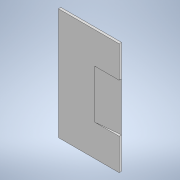
# Autodesk Inventor part: Stage
Saved by Autodesk Inventor 2021 (Build 250183000, 183)
## iProperties
Created: 2022-07-02
Part Number: Stage
Material: 一般
Document SubType Name: Modeling
Designer: tazak
Density: 1 g/cm^3
Appearance: 既定
Author: tazak
Autodesk Inventor part; units mm, degrees
ref_plane "YZ Plane" through (0, 0, 0) normal (1, 0, 0) x (0, 1, 0)
ref_plane "XZ Plane" through (0, 0, 0) normal (0, 1, 0) x (-1, 0, 0)
ref_plane "XY Plane" through (0, 0, 0) normal (0, 0, 1) x (1, 0, 0)
sketch "スケッチ1" plane through (0, 0, 0) normal (0, 0, 1) x (1, 0, 0)
  line L0 (-800, 2300) -> (1700, 2300)
  line L1 (1700, 2300) -> (1700, -2300)
  line L2 (1700, -2300) -> (-800, -2300)
  line L3 (-800, -2300) -> (-800, 2300)
  line L4 (-1000, 2500) -> (2000, 2500) construction
  line L5 (2000, 2500) -> (2000, -2500) construction
  line L6 (2000, -2500) -> (-1000, -2500) construction
  line L7 (-1000, -2500) -> (-1000, 2500) construction
  point P0 (0, 0)
  point P1 (-1000, 0)
  dimension "d13" = 2500
  dimension "d14" = 5000
  dimension "d15" = 1000
  dimension "d16" = 2000
  dimension "d17" = 200
  dimension "d18" = 200
  dimension "d19" = 200
  constraints: 16 end point, 4 parallel, 2 horizontal, 2 perpendicular, 1 horizontal alignment, 1 midpoint
  measures "d13" distance of L0.start L0.end
  measures "d14" distance of L6.end L4.start
  measures "d15" distance from line of point (0, 0) L7
  measures "d16" distance from line of L5 point (0, 0)
  measures "d17" distance between parallel lines of L3 L7
  measures "d18" distance between parallel lines of L4 L0
  measures "d19" distance between parallel lines of L6 L2
extrude "押し出し1" add sketch "スケッチ1" along normal blind 100
sketch "スケッチ4" plane through (0, 0, 0) normal (0, 1, 0) x (-1, 0, 0)
  line L0 (-1700, 0) -> (-700, 100)
  line L1 (-1700, 100) -> (800, 100) projected
  line L2 (-1700, 0) -> (-1700, 100) projected
  line L3 (-700, 100) -> (-1700, 100)
  line L4 (-1700, 100) -> (-1700, 0)
  point P0 (0, 0)
  dimension "d20" = 1000
  constraints: 6 end point, 2 perpendicular, 1 point on line
  measures "d20" horizontal distance of L0.start L0.end
extrude "押し出し4" cut sketch "スケッチ4" along normal mid plane 2000
